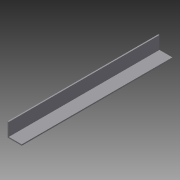
# Autodesk Inventor part: 16in 2inL
Saved by Autodesk Inventor 2015 (Build 190159000, 159)
## iProperties
Created: 2017-01-05
Part Number: 16in 2inL
Material: Generic
Document SubType Name: Modeling
Designer: ps2du
Density: 1 g/cm^3
Appearance: Default
Author: ps2du
Autodesk Inventor part; units mm, degrees
ref_plane "YZ Plane" through (0, 0, 0) normal (1, 0, 0) x (0, 1, 0)
ref_plane "XZ Plane" through (0, 0, 0) normal (0, 1, 0) x (-1, 0, 0)
ref_plane "XY Plane" through (0, 0, 0) normal (0, 0, 1) x (1, 0, 0)
sketch "Sketch1" plane through (0, 0, 0) normal (0, 0, 1) x (1, 0, 0)
  line L0 (0, 0) -> (38.1, 0)
  line L1 (38.1, 0) -> (38.1, 3.175)
  line L2 (38.1, 3.175) -> (0, 3.175)
  line L3 (0, 3.175) -> (0, 0)
  dimension "d0" = 38.1
  dimension "d1" = 3.175
  constraints: 8 end point, 2 parallel, 1 horizontal, 1 perpendicular
  measures "d0" distance of L2.end L1.end
  measures "d1" distance between parallel lines of L0 L2
extrude "Extrusion1" add sketch "Sketch1" along normal blind 355.6
sketch "Sketch2" plane through (0, 0, 355.6) normal (0, 0, 1) x (1, 0, 0)
  line L0 (0, 0) -> (3.175, 0)
  line L1 (3.175, 0) -> (3.175, 38.1)
  line L2 (3.175, 38.1) -> (0, 38.1)
  line L3 (0, 38.1) -> (0, 0)
  dimension "d4" = 3.175
  dimension "d5" = 38.1
  constraints: 8 end point, 2 parallel, 1 horizontal, 1 perpendicular
  measures "d4" distance of L2.end L1.end
  measures "d5" distance between parallel lines of L0 L2
extrude "Extrusion2" add sketch "Sketch2" against normal blind 355.6
sketch "Sketch3" plane through (0, 0, 355.6) normal (0, 0, 1) x (1, 0, 0)
  line L0 (0, 0) -> (38.1, 0)
  line L1 (38.1, 0) -> (38.1, 3.175)
  line L2 (38.1, 3.175) -> (3.175, 3.175)
  line L3 (38.1, 3.175) -> (3.175, 3.175) projected
  line L4 (3.175, 3.175) -> (3.175, 38.1)
  line L5 (3.175, 38.1) -> (0, 38.1)
  line L6 (0, 38.1) -> (0, 0)
  line L7 (0, 38.1) -> (0, 0) projected
  constraints: 12 end point, 3 perpendicular, 2 collinear, 1 horizontal
extrude "Extrusion3" add sketch "Sketch3" along normal blind 50.8
body "Solid1"
